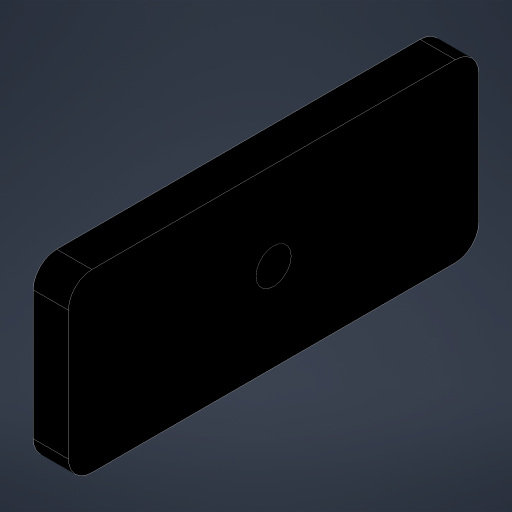
# Autodesk Inventor part: Plate
Saved by Autodesk Inventor 2023.2 (Build 272271030, 271C)
## iProperties
Created: 2023-04-07
Part Number: Plate
Material: Generic
Document SubType Name: Modeling
Designer: Elias Braun
Density: 1 g/cm^3
Appearance: Default
Author: Elias Braun
Autodesk Inventor part; units mm, degrees
ref_plane "YZ Plane" through (0, 0, 0) normal (1, 0, 0) x (0, 1, 0)
ref_plane "XZ Plane" through (0, 0, 0) normal (0, 1, 0) x (-1, 0, 0)
ref_plane "XY Plane" through (0, 0, 0) normal (0, 0, 1) x (1, 0, 0)
sketch "Sketch1" plane through (0, 0, 0) normal (1, 0, 0) x (0, 1, 0)
  circle A0 centre (0, 0) radius 1.5
  line L0 (-7.5, 17.5) -> (-7.5, -17.5)
  line L1 (-7.5, -17.5) -> (7.5, -17.5)
  line L2 (7.5, -17.5) -> (7.5, 17.5)
  line L3 (7.5, 17.5) -> (-7.5, 17.5)
  line L4 (-7.5, 17.5) -> (7.5, -17.5) construction
  line L5 (-7.5, -17.5) -> (7.5, 17.5) construction
  dimension "d0" = 3
  dimension "d1" = 35
  dimension "d2" = 15
  constraints: 12 end point, 2 midpoint, 2 parallel, 1 centre point, 1 coincident, 1 perpendicular, 1 vertical
  measures "d0" diameter of A0
  measures "d1" distance of L0.start L0.end
  measures "d2" distance of L1.end L0.end
extrude "Extrusion1" add sketch "Sketch1" along normal blind 3
fillet "Fillet1" radius 2 4 edges at (1.5, 7.5, 17.5) (1.5, -7.5, 17.5) (1.5, -7.5, -17.5) (1.5, 7.5, -17.5)
body "Solid1"
